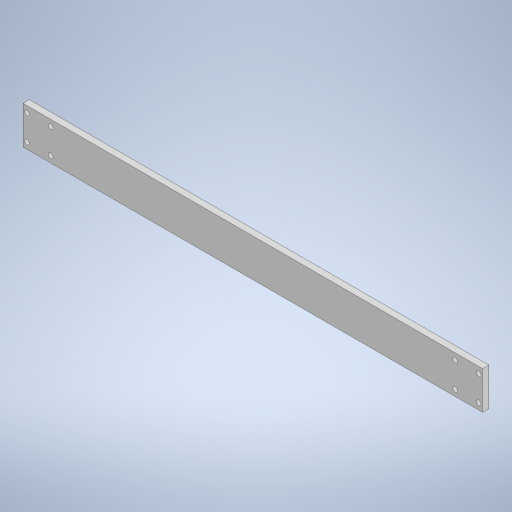
# Autodesk Inventor part: центр_рейка
Saved by Autodesk Inventor 2023.1 (Build 271208000, 208)
## iProperties
Created: 2025-12-22
Part Number: центр_рейка
Material: Типовые
Document SubType Name: Modeling
Designer: DELL
Density: 1 g/cm^3
Appearance: По умолчанию
Author: DELL
Autodesk Inventor part; units mm, degrees
ref_plane "YZ Plane" through (0, 0, 0) normal (1, 0, 0) x (0, 1, 0)
ref_plane "XZ Plane" through (0, 0, 0) normal (0, 1, 0) x (-1, 0, 0)
ref_plane "XY Plane" through (0, 0, 0) normal (0, 0, 1) x (1, 0, 0)
sketch "Эскиз1" plane through (0, 0, 0) normal (0, 0, 1) x (1, 0, 0)
  circle A0 centre (-7.5, -22.95) radius 1.5 projected
  circle A1 centre (7.5, -22.95) radius 1.5 projected
  circle A2 centre (7.5, -6.95) radius 1.5 projected
  circle A3 centre (-7.5, -6.95) radius 1.5 projected
  line L0 (-281.4, -2.95) -> (10, -2.95)
  line L1 (10, -2.95) -> (10, -26.95)
  line L2 (10, -26.95) -> (-281.4, -26.95)
  line L3 (-281.4, -26.95) -> (-281.4, -2.95)
  line L4 (-281.4, -2.95) -> (10, -26.95) construction
  line L5 (10, -2.95) -> (-281.4, -26.95) construction
  line L6 (-135.7, -14.95) -> (-135.7, -26.95) construction
  circle A4 centre (-263.9, -22.95) radius 1.5
  circle A5 centre (-278.9, -22.95) radius 1.5
  circle A6 centre (-278.9, -6.95) radius 1.5
  circle A7 centre (-263.9, -6.95) radius 1.5
  point P0 (0, 0)
  dimension "d5" = 291.4
  dimension "d8" = 2.5
  dimension "d9" = 4
  dimension "d10" = 4
  constraints: 14 end point, 4 centre point, 4 symmetric about line, 3 midpoint, 2 parallel, 1 horizontal, 1 perpendicular, 4 other
  measures "d5" distance of L1.end L2.end
  measures "d8" distance from line of L1 A2.centre
  measures "d9" distance from line of L0 A2.centre
  measures "d10" distance from line of L2 A0.centre
extrude "Выдавливание1" add sketch "Эскиз1" along normal blind 4
